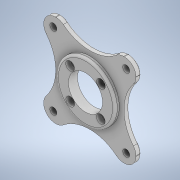
# Autodesk Inventor part: worm gear mountV2
Saved by Autodesk Inventor 2021 (Build 250183000, 183)
## iProperties
Created: 2020-04-08
Part Number: worm gear mountV2
Material: Generic
Document SubType Name: Modeling
Designer: User01
Density: 1 g/cm^3
Appearance: Default
Author: User01
Autodesk Inventor part; units mm, degrees
ref_plane "YZ Plane" through (0, 0, 0) normal (1, 0, 0) x (0, 1, 0)
ref_plane "XZ Plane" through (0, 0, 0) normal (0, 1, 0) x (-1, 0, 0)
ref_plane "Work Plane1" through (0, 0, 3) normal (0, 0, 1) x (1, 0, 0)
sketch "Sketch3" plane through (0, 0, 3) normal (0, 0, 1) x (1, 0, 0)
  circle A0 centre (21, -21) radius 19
  point P0 (0, 0)
  dimension "d68" = 38
  constraints: 1 centre point
  measures "d68" diameter of A0
sketch "Sketch1" plane through (0, 0, 0) normal (0, 0, 1) x (1, 0, 0)
  circle A0 centre (21.0028, -21) radius 11
  line L0 (0.1013, -0.0126) -> (42.0187, 0.0702) construction
  line L1 (42.0187, 0.0702) -> (42.1019, -42.0132) construction
  line L2 (42.1019, -42.0132) -> (0.1845, -42.096) construction
  line L3 (0.1845, -42.096) -> (0.1013, -0.0126) construction
  circle A1 centre (-2.5, 2.4173) radius 2.25
  circle A2 centre (44.5, 2.5) radius 2.25
  circle A3 centre (44.5056, -44.5634) radius 2.25
  circle A4 centre (-2.4944, -44.5827) radius 2.25
  circle A5 centre (11.0885, -11.1125) radius 1.75
  circle A6 centre (30.876, -30.923) radius 1.75
  circle A7 centre (30.9911, -11.2198) radius 1.75
  circle A8 centre (11.1918, -30.965) radius 1.75
  line L4 (0.25, -41.5175) -> (0.25, -42.0959)
  line L5 (-3.9442, -21.0833) -> (49.9388, -21.0612) construction
  line L6 (-3.9442, -21.0833) -> (49.9388, -21.0833) construction
  line L7 (21.0062, -49.0438) -> (20.9993, 8.8375) construction
  line L8 (21.0028, -21) -> (45.1212, -21) construction
  circle A9 centre (21.0028, -21) radius 22 construction
  line L9 (-16.2433, -1.8185) -> (66.6553, -1.8185) construction
  line L10 (-11.573, -40.0827) -> (64.3978, -40.0827) construction
  line L11 (-11.573, -40.0827) -> (64.3978, -40.0827) construction
  line L12 (2.0001, 8.8375) -> (1.9996, -51.4762) construction
  line L13 (2.0001, 8.8375) -> (62.3138, 8.8375) construction
  line L14 (40, 9.446) -> (40.0004, -50.8134) construction
  line L15 (40, 9.446) -> (100.1505, 9.446) construction
  line L16 (-8.75, 8.6673) -> (50.75, 8.6673)
  line L17 (50.75, 8.6673) -> (50.75, -50.8134)
  line L18 (50.75, -50.8134) -> (-8.75, -50.8134)
  line L19 (-8.75, -50.8134) -> (-8.75, 8.6673)
  arc A10 (2.0001, 8.6673) -> (40, 8.6673) centre (21, 28.3163) ccw
  arc A11 (-8.75, -40.0827) -> (-8.75, -1.8185) centre (-28.4787, -20.9506) ccw
  arc A12 (50.75, -1.8185) -> (50.75, -40.0827) centre (70.5001, -20.9506) ccw
  arc A13 (40.0004, -50.8134) -> (1.9996, -50.8134) centre (21, -70.009) ccw
  point P0 (0, 0)
  dimension "d2" = 22
  dimension "d8" = 3.5
  dimension "d9" = 3.5
  dimension "d10" = 3.5
  dimension "d11" = 3.5
  dimension "d71" = 23.5
  dimension "d72" = 23.5
  dimension "d74" = 23.5
  dimension "d75" = 23.5
  dimension "d76" = 23.5
  dimension "d77" = 23.5
  dimension "d78" = 23.5
  dimension "d79" = 23.5
  dimension "d98" = 44
  dimension "d103" = 4.5
  dimension "d106" = 4.5
  dimension "d107" = 4.5
  dimension "d121" = 4.5
  dimension "d122" = 4.5
  dimension "d123" = 4.5
  dimension "d124" = 4.5
  dimension "d126" = 4
  dimension "d129" = 4
  dimension "d131" = 4
  dimension "d132" = 4
  constraints: 34 end point, 18 point on line, 14 centre point, 8 point on circle, 7 horizontal, 3 equal length, 2 parallel, 1 coincident, 1 perpendicular, 3 other
  measures "d2" diameter of A0
  measures "d8" diameter of A5
  measures "d9" diameter of A6
  measures "d10" diameter of A7
  measures "d11" diameter of A8
  measures "d71" distance from line of L5 A1.centre
  measures "d72" distance from line of L5 A4.centre
  measures "d74" distance from line of L7 A2.centre
  measures "d75" distance from line of L7 A3.centre
  measures "d76" distance from line of L8 A2.centre
  measures "d77" distance from line of L5 A3.centre
  measures "d78" distance from line of L7 A1.centre
  measures "d79" distance from line of L7 A4.centre
  measures "d98" diameter of A9
  measures "d103" distance from line of A4.centre L11
  measures "d106" distance from line of A2.centre L14
  measures "d107" distance from line of A1.centre L12
  measures "d121" diameter of A1
  measures "d122" diameter of A2
  measures "d123" diameter of A3
  measures "d124" diameter of A4
  measures "d126" distance edge to line of A1 L16
  measures "d129" distance edge to line of A3 L18
  measures "d131" distance edge to line of A2 L17
  measures "d132" distance edge to line of A1 L19
extrude "Extrusion1" add sketch "Sketch1" along normal blind 3 contours L16 A10 L17 A12 L18 A13 L19 A11
extrude "Extrusion3" add sketch "Sketch3" along normal blind 2.8
sketch "Sketch2" plane through (0, 0, 3) normal (0, 0, 1) x (1, 0, 0)
  circle A0 centre (11.1918, -30.965) radius 1.75 projected
  circle A1 centre (11.1918, -30.965) radius 2.825
  circle A2 centre (11.0885, -11.1125) radius 1.75 projected
  circle A3 centre (11.0885, -11.1125) radius 2.825
  circle A4 centre (30.876, -30.923) radius 1.75 projected
  circle A5 centre (30.876, -30.923) radius 2.825
  circle A6 centre (30.9911, -11.2198) radius 1.75 projected
  circle A7 centre (30.9911, -11.2198) radius 2.825
  point P0 (0, 0)
  dimension "d59" = 5.65
  dimension "d60" = 5.65
  dimension "d61" = 5.65
  dimension "d62" = 5.65
  constraints: 4 centre point, 4 coincident
  measures "d59" diameter of A1
  measures "d60" diameter of A3
  measures "d61" diameter of A5
  measures "d62" diameter of A7
extrude "Extrusion2" cut sketch "Sketch2" along normal blind 3 and the other way blind 0.5 contours A0 | A1 | A2 | A3 | A4 | A5 | A6 | A7
thicken "Thicken1" operation add thickness 3 both sides no extend neighbours yes toward (0, 0, 1) faces at (24.4564, -21, 3)
fillet "Fillet2" radius 0.5 12 edges at (45.3752, -50.8134, 0) (21, -43, 0) (-3.3752, -50.8134, 0) (-8.75, -45.448, 0) (-0.9967, -20.9506, 0) (-8.75, 3.4244, 0) (-3.375, 8.6673, 0) (21, 0.9835, 0) (45.375, 8.6673, 0) (50.75, 3.4244, 0) (43.0028, -20.9506, 0) (50.75, -45.448, 0)
fillet "Fillet2" radius 1.5 1 edges at (2, -21, 5.8)
fillet "Fillet2" radius 7.5 12 edges at (2.0001, 8.6673, 1.5) (40, 8.6673, 1.5) (50.75, 8.6673, 1.5) (50.75, -1.8185, 1.5) (50.75, -40.0827, 1.5) (50.75, -50.8134, 1.5) (40.0004, -50.8134, 1.5) (1.9996, -50.8134, 1.5) (-8.75, -50.8134, 1.5) (-8.75, -40.0827, 1.5) (-8.75, -1.8185, 1.5) (-8.75, 8.6673, 1.5)
body "Solid1"
